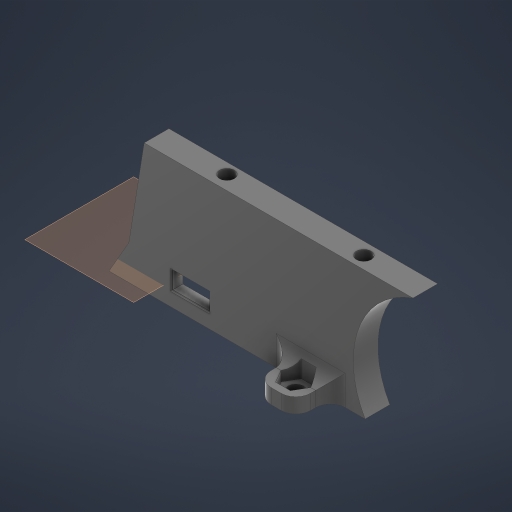
# Autodesk Inventor part: bok_lewy
Saved by Autodesk Inventor 2024 (Build 280153000, 153)
## iProperties
Created: 2024-05-25
Part Number: bok_lewy
Material: ABS Plastic
Document SubType Name: Modeling
Designer: Adam
Density: 1.06 g/cm^3
Appearance: Smooth - White
Mass: 4.70038 g
Surface Area: 30.9781 cm^2
Volume: 4.70038 cm^3
Author: Adam
Autodesk Inventor part; units mm, degrees
ref_plane "YZ Plane" through (0, 0, 0) normal (1, 0, 0) x (0, 1, 0)
ref_plane "XZ Plane" through (0, 0, 0) normal (0, 1, 0) x (-1, 0, 0)
ref_plane "XY Plane" through (0, 0, 0) normal (0, 0, 1) x (1, 0, 0)
sketch "Sketch1" plane through (0, 0, 0) normal (0, 0, 1) x (1, 0, 0)
  line L0 (61.4575, 26) -> (7.1245, 26)
  line L1 (7.1245, 26) -> (4.1002, 7.362)
  line L2 (51.7851, 0) -> (0, 0)
  line L3 (0, 0) -> (3.8581, 6.6824)
  arc A0 (61.4575, 26) -> (51.7851, 0) centre (67.3735, 9) ccw
  arc A1 (3.8581, 6.6824) -> (4.1002, 7.362) centre (2.126, 7.6824) ccw
  constraints: 8 end point, 4 point on circle, 2 centre point, 1 horizontal
extrude "Extrusion1" add sketch "Sketch1" along normal blind 5
ref_plane "Work Plane1" through (0, 3, 0) normal (0, 1, 0) x (1, 0, 0)
sketch "Sketch6" plane through (0, 0, 0) normal (0, 0, -1) x (-1, 0, 0)
  line L0 (-20.4243, 6.6958) -> (-12.4243, 6.6958)
  line L1 (-12.4243, 6.6958) -> (-12.4243, 2.6958)
  line L2 (-12.4243, 2.6958) -> (-20.4243, 2.6958)
  line L3 (-20.4243, 2.6958) -> (-20.4243, 6.6958)
  line L4 (-20.4243, 6.6958) -> (-12.4243, 2.6958) construction
  line L5 (-12.4243, 6.6958) -> (-20.4243, 2.6958) construction
  point P0 (-18.6243, 3.4939)
  point P1 (-18.6263, 5.8939)
  point P2 (-14.2243, 5.8977)
  point P3 (-14.2243, 3.4977)
  point P4 (-16.4243, 4.6958)
  dimension "d52" = 8
  dimension "d53" = 4
  constraints: 12 end point, 2 midpoint, 2 parallel, 1 horizontal, 1 perpendicular
  measures "d52" distance of L1.end L2.end
  measures "d53" distance of L0.end L1.end
extrude "Extrusion6" cut sketch "Sketch6" against normal through all
chamfer "Chamfer2" distance 2.5 distance2 4.5 4 edges at (16.4243, 6.6958, 0) (20.4243, 4.6958, 0) (16.4243, 2.6958, 0) (12.4243, 4.6958, 0) measured on face at (16.4243, 2.1958, 0) measured on face at (20.9243, 4.6958, 0) measured on face at (16.4243, 7.1958, 0) measured on face at (11.9243, 4.6958, 0)
sketch "Sketch9" plane through (0, 0, 0) normal (0, 0, -1) x (-1, 0, 0)
  line L0 (-46.6305, 22.9528) -> (-16.175, 22.9528) construction
  line L1 (-16.175, 22.9528) -> (-16.175, 16.5958) construction
  line L2 (-16.175, 16.5958) -> (-46.6305, 16.5958) construction
  line L3 (-46.6305, 16.5958) -> (-46.6305, 22.9528) construction
  line L4 (-39.7692, 16.7243) -> (-41.2918, 16.7243)
  line L5 (-41.2918, 16.7243) -> (-41.2918, 20.7679)
  line L6 (-41.2918, 20.7679) -> (-42.3991, 18.1579)
  line L7 (-42.3991, 18.1579) -> (-43.447, 18.1579)
  line L8 (-43.447, 18.1579) -> (-44.5543, 20.7679)
  line L9 (-44.5543, 20.7679) -> (-44.5543, 16.7243)
  line L10 (-44.5543, 16.7243) -> (-45.9978, 16.7243)
  line L11 (-45.9978, 16.7243) -> (-45.9978, 22.8243)
  line L12 (-45.9978, 22.8243) -> (-44.233, 22.8243)
  line L13 (-44.233, 22.8243) -> (-42.8786, 19.8139)
  line L14 (-42.8786, 19.8139) -> (-41.534, 22.8243)
  line L15 (-41.534, 22.8243) -> (-39.7692, 22.8243)
  line L16 (-39.7692, 22.8243) -> (-39.7692, 16.7243)
  line L17 (-38.5038, 16.7243) -> (-38.5038, 22.8243)
  line L18 (-38.5038, 22.8243) -> (-34.3811, 22.8243)
  line L19 (-34.3811, 22.8243) -> (-34.3811, 21.6626)
  line L20 (-34.3811, 21.6626) -> (-36.9812, 21.6626)
  line L21 (-36.9812, 21.6626) -> (-36.9812, 20.59)
  line L22 (-36.9812, 20.59) -> (-34.5837, 20.59)
  line L23 (-34.5837, 20.59) -> (-34.5837, 19.4283)
  line L24 (-34.5837, 19.4283) -> (-36.9812, 19.4283)
  line L25 (-36.9812, 19.4283) -> (-36.9812, 17.886)
  line L26 (-36.9812, 17.886) -> (-34.3811, 17.886)
  line L27 (-34.3811, 17.886) -> (-34.3811, 16.7243)
  line L28 (-34.3811, 16.7243) -> (-38.5038, 16.7243)
  line L29 (-29.2598, 21.6626) -> (-31.8205, 21.6626)
  line L30 (-31.8205, 21.6626) -> (-31.8205, 20.5109)
  line L31 (-31.8205, 20.5109) -> (-29.4625, 20.5109)
  line L32 (-29.4625, 20.5109) -> (-29.4625, 19.3492)
  line L33 (-29.4625, 19.3492) -> (-31.8205, 19.3492)
  line L34 (-31.8205, 19.3492) -> (-31.8205, 16.7243)
  line L35 (-31.8205, 16.7243) -> (-33.343, 16.7243)
  line L36 (-33.343, 16.7243) -> (-33.343, 22.8243)
  line L37 (-33.343, 22.8243) -> (-29.2598, 22.8243)
  line L38 (-29.2598, 22.8243) -> (-29.2598, 21.6626)
  spline S0 degree 2 poles (-22.9176, 19.7743) (-22.9176, 18.2913) (-24.4995, 16.5958) (-25.8737, 16.5958) knots 0 0 0 1 2 2 2
  spline S1 degree 2 poles (-25.8737, 16.5958) (-27.2529, 16.5958) (-28.8248, 18.3111) (-28.8248, 19.7743) knots 0 0 0 1 2 2 2
  spline S2 degree 2 poles (-28.8248, 19.7743) (-28.8248, 21.2425) (-27.2529, 22.9528) (-25.8737, 22.9528) knots 0 0 0 1 2 2 2
  spline S3 degree 2 poles (-25.8737, 22.9528) (-24.4995, 22.9528) (-22.9176, 21.2524) (-22.9176, 19.7743) knots 0 0 0 1 2 2 2
  spline S4 degree 2 poles (-24.4995, 19.7743) (-24.4995, 20.323) (-24.7219, 21.0892) (-24.9147, 21.3314) knots 0 0 0 1 2 2 2
  spline S5 degree 2 poles (-24.9147, 21.3314) (-25.1075, 21.5836) (-25.6018, 21.8011) (-25.8688, 21.8011) knots 0 0 0 1 2 2 2
  spline S6 degree 2 poles (-25.8688, 21.8011) (-26.1505, 21.8011) (-26.6102, 21.5984) (-26.8228, 21.3413) knots 0 0 0 1 2 2 2
  spline S7 degree 2 poles (-26.8228, 21.3413) (-27.0107, 21.1041) (-27.243, 20.3181) (-27.243, 19.7743) knots 0 0 0 1 2 2 2
  spline S8 degree 2 poles (-27.243, 19.7743) (-27.243, 19.2108) (-27.0205, 18.4693) (-26.8277, 18.2172) knots 0 0 0 1 2 2 2
  spline S9 degree 2 poles (-26.8277, 18.2172) (-26.635, 17.9651) (-26.1357, 17.7476) (-25.8688, 17.7476) knots 0 0 0 1 2 2 2
  spline S10 degree 2 poles (-25.8688, 17.7476) (-25.5969, 17.7476) (-25.0927, 17.9799) (-24.9098, 18.2271) knots 0 0 0 1 2 2 2
  spline S11 degree 2 poles (-24.9098, 18.2271) (-24.712, 18.494) (-24.4995, 19.2009) (-24.4995, 19.7743) knots 0 0 0 1 2 2 2
  line L39 (-16.783, 16.7243) -> (-18.2561, 16.7243)
  line L40 (-18.2561, 16.7243) -> (-20.6091, 20.9755)
  line L41 (-20.6091, 20.9755) -> (-20.6091, 16.7243)
  line L42 (-20.6091, 16.7243) -> (-22.0081, 16.7243)
  line L43 (-22.0081, 16.7243) -> (-22.0081, 22.8243)
  line L44 (-22.0081, 22.8243) -> (-20.1296, 22.8243)
  line L45 (-20.1296, 22.8243) -> (-18.182, 19.3294)
  line L46 (-18.182, 19.3294) -> (-18.182, 22.8243)
  line L47 (-18.182, 22.8243) -> (-16.783, 22.8243)
  line L48 (-16.783, 22.8243) -> (-16.783, 16.7243)
  point P0 (0, 0)
  constraints: 2 other
emboss "Emboss1" sketch "Sketch9" operation cut depth 1 direction (0, 0, 1)
sketch "Sketch10" plane through (0, 0, 0) normal (0, -1, 0) x (1, 0, 0)
  line L0 (44.7851, 12) -> (44.7851, 5) projected
  line L1 (36.7851, 12) -> (44.7851, 12) projected
  circle A0 centre (40.7851, 8) radius 1.55 projected
  line L2 (44.7851, 5) -> (36.7851, 5)
  line L3 (36.7851, 5) -> (36.7851, 12)
  line L4 (36.7851, 12) -> (44.7851, 12)
  line L5 (44.7851, 12) -> (44.7851, 5)
  circle A1 centre (40.7851, 8) radius 1.55
  point P0 (0, 0)
  constraints: 8 end point, 2 parallel, 1 centre point, 1 coincident, 1 concentric, 1 horizontal, 1 perpendicular
extrude "Extrusion8" add sketch "Sketch10" against normal blind 3
sketch "Sketch11" plane through (7.1245, 26, 0) normal (0, 1, 0) x (1, 0, 0)
  circle A0 centre (13.8867, -2.162) radius 1.5 projected
  circle A1 centre (41.8867, -2.5) radius 1.5 projected
  circle A2 centre (41.8867, -2.5) radius 1.5
  circle A3 centre (13.8867, -2.162) radius 1.5
  point P0 (-7.1245, 0)
  constraints: 2 centre point, 2 coincident, 2 concentric
extrude "Extrusion9" cut sketch "Sketch11" against normal blind 2
sketch "Sketch12" plane through (0, 3, 0) normal (0, 1, 0) x (1, 0, 0)
  circle A0 centre (40.7851, -8) radius 1.55 projected
  line L0 (42.2876, -5.3976) -> (43.7901, -8) projected
  line L1 (43.7901, -8) -> (42.2876, -10.6024) projected
  line L2 (42.2876, -10.6024) -> (39.2826, -10.6024) projected
  line L3 (39.2826, -10.6024) -> (37.7801, -8) projected
  line L4 (37.7801, -8) -> (39.2826, -5.3976) projected
  line L5 (39.2826, -5.3976) -> (42.2876, -5.3976) projected
  line L6 (43.7901, -8) -> (42.2876, -10.6024)
  line L7 (42.2876, -10.6024) -> (39.2826, -10.6024)
  line L8 (39.2826, -10.6024) -> (37.7801, -8)
  line L9 (37.7801, -8) -> (39.2826, -5.3976)
  line L10 (39.2826, -5.3976) -> (42.2876, -5.3976)
  line L11 (42.2876, -5.3976) -> (43.7901, -8)
  circle A1 centre (40.7851, -8) radius 1.55
  point P0 (0, 0)
  constraints: 12 end point, 2 coincident, 1 centre point, 1 concentric, 13 other
extrude "Extrusion10" cut sketch "Sketch12" against normal blind 2
fillet "Fillet5" radius 3 4 edges at (44.7851, 1.5, 12) (44.7851, 1.5, 5) (36.7851, 1.5, 12) (36.7851, 1.5, 5)
fillet "Fillet6" radius 3 3 edges at (35.2851, 3, 5) (40.7851, 3, 5) (46.2851, 3, 5)
body "Solid1"
